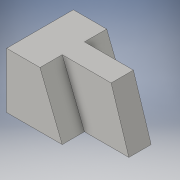
# Autodesk Inventor part: Figure 7_28_1
Saved by Autodesk Inventor 2016 (Build 200138000, 138)
## iProperties
Created: 2016-07-19
Part Number: Figure 7_28_1
Material: Generic
Document SubType Name: Modeling
Designer: cfkguest
Density: 1 g/cm^3
Appearance: Default
Author: cfkguest
Autodesk Inventor part; units mm, degrees
ref_plane "YZ Plane" through (0, 0, 0) normal (1, 0, 0) x (0, 1, 0)
ref_plane "XZ Plane" through (0, 0, 0) normal (0, 1, 0) x (-1, 0, 0)
ref_plane "XY Plane" through (0, 0, 0) normal (0, 0, 1) x (1, 0, 0)
sketch "Sketch1" plane through (0, 0, 0) normal (0, 0, 1) x (1, 0, 0)
  line L0 (-20.4911, 10.9492) -> (11.2589, 10.9492)
  line L1 (11.2589, 10.9492) -> (11.2589, -20.8008)
  line L2 (11.2589, -20.8008) -> (-20.4911, -20.8008)
  line L3 (-20.4911, -20.8008) -> (-20.4911, 10.9492)
  point P0 (0, 0)
  dimension "d0" = 31.75
  dimension "d1" = 31.75
  constraints: 8 end point, 2 parallel, 1 horizontal, 1 perpendicular
  measures "d0" distance of L0.start L0.end
  measures "d1" distance of L0.end L1.end
extrude "Extrusion1" add sketch "Sketch1" along normal blind 38.1
sketch "Sketch2" plane through (0, 0, 38.1) normal (0, 0, 1) x (1, 0, 0)
  line L0 (-20.4911, -20.8008) -> (11.2589, -20.8008) projected
  line L1 (11.2589, -20.8008) -> (-1.4411, 10.9492)
  line L2 (11.2589, 10.9492) -> (-20.4911, 10.9492) projected
  line L3 (-1.4411, 10.9492) -> (11.2589, 10.9492)
  line L4 (11.2589, -20.8008) -> (11.2589, 10.9492) projected
  line L5 (11.2589, 10.9492) -> (11.2589, -20.8008)
  point P0 (0, 0)
  dimension "d4" = 19.05
  constraints: 6 end point, 2 collinear, 1 point on line
  measures "d4" distance of L2.end L1.end
sketch "Sketch3" plane through (11.2589, -20.8008, 0) normal (1, 0, 0) x (0, 0, -1)
  line L0 (0, 31.75) -> (-38.1, 31.75) projected
  line L1 (0, 0) -> (-38.1, 0) projected
  line L2 (-25.4, 31.75) -> (-12.7, 31.75)
  line L3 (-12.7, 31.75) -> (-12.7, 0)
  line L4 (-12.7, 0) -> (-25.4, 0)
  line L5 (-25.4, 0) -> (-25.4, 31.75)
  line L6 (0, 31.75) -> (0, 0) projected
  line L7 (-38.1, 0) -> (-38.1, 31.75) projected
  point P0 (0, 20.8008)
  dimension "d5" = 12.7
  dimension "d6" = 12.7
  constraints: 8 end point, 2 parallel, 2 point on line, 1 horizontal, 1 perpendicular
  measures "d5" distance between parallel lines of L6 L3
  measures "d6" distance between parallel lines of L7 L5
extrude "Extrusion2" add sketch "Sketch3" along normal blind 25.4 contours L3 L1 L5 L0
sketch "Sketch4" plane through (11.2589, -20.8008, 25.4) normal (0, 0, 1) x (1, 0, 0)
  line L0 (0, 0) -> (25.4, 0) projected
  line L1 (25.4, 0) -> (15.2492, 31.75)
  line L2 (0, 31.75) -> (25.4, 31.75) projected
  line L3 (15.2492, 31.75) -> (25.4, 31.75)
  line L4 (25.4, 31.75) -> (25.4, 0) projected
  line L5 (25.4, 31.75) -> (25.4, 0)
  point P0 (-11.2589, 20.8008)
  constraints: 6 end point, 1 collinear, 1 perpendicular, 1 point on line
extrude "Extrusion3" cut sketch "Sketch4" against normal blind 25.4
extrude "Extrusion4" cut sketch "Sketch2" against normal blind 12.7
sketch "Sketch5" plane through (0, 0, 0) normal (0, 0, -1) x (-1, 0, 0)
  line L0 (-11.2589, 10.9492) -> (-11.2589, -20.8008) projected
  line L1 (-11.2589, -20.8008) -> (1.4411, 10.9492) projected
  line L2 (-11.2589, -20.8008) -> (1.4411, 10.9492)
  line L3 (20.4911, 10.9492) -> (-11.2589, 10.9492) projected
  line L4 (1.4411, 10.9492) -> (-11.2589, 10.9492)
  line L5 (-11.2589, 10.9492) -> (-11.2589, -20.8008)
  point P0 (0, 0)
  constraints: 6 end point, 2 collinear, 1 perpendicular
extrude "Extrusion5" cut sketch "Sketch5" against normal blind 12.7
body "Solid1"
